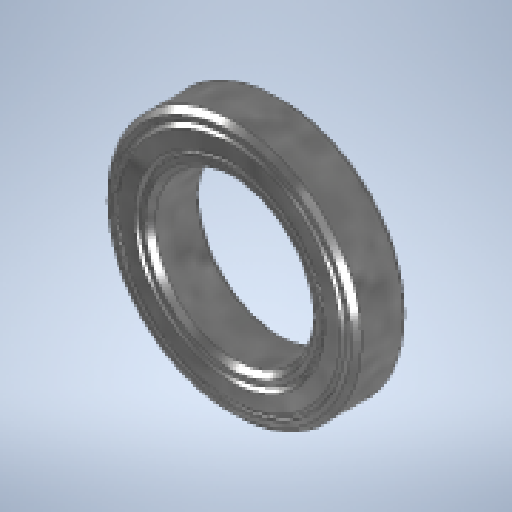
# Autodesk Inventor part: 6203베어링
Saved by Autodesk Inventor 2023 (Build 270158000, 158)
## iProperties
Created: 2022-06-08
Part Number: 6203베어링
Material: 일반
Document SubType Name: Modeling
Designer: fly01
Density: 1 g/cm^3
Appearance: 기본값
Author: fly01
Autodesk Inventor part; units mm, degrees
ref_plane "YZ Plane" through (0, 0, 0) normal (1, 0, 0) x (0, 1, 0)
ref_plane "XZ Plane" through (0, 0, 0) normal (0, 1, 0) x (-1, 0, 0)
ref_plane "XY Plane" through (0, 0, 0) normal (0, 0, 1) x (1, 0, 0)
sketch "스케치1" plane through (0, 0, 0) normal (0, 0, 1) x (1, 0, 0)
  circle A0 centre (0, 0) radius 7.5
  circle A1 centre (0, 0) radius 12
  dimension "d0" = 15
  dimension "d1" = 24
  constraints: 2 centre point, 2 coincident
  measures "d0" diameter of A0
  measures "d1" diameter of A1
extrude "돌출1" add sketch "스케치1" along normal mid plane 5
chamfer "모따기1" distance 0.5 angle 45 4 edges at (-12, 0, 2.5) (-12, 0, -2.5) (-7.5, 0, 2.5) (-7.5, 0, -2.5)
sketch "스케치2" plane through (0, 0, 0) normal (0, 1, 0) x (-1, 0, 0)
  line L0 (-11.5, 2.5) -> (11.5, 2.5) projected
  line L1 (11, 2.5) -> (11, 2.2414)
  line L2 (10.8293, 2.1707) -> (10.5, 2.5)
  line L3 (12, 0) -> (7.5, 0)
  line L4 (7.5, 2) -> (7.5, -2) projected
  arc A0 (10.8293, 2.1707) -> (11, 2.2414) centre (10.9, 2.2414) ccw
  line L5 (9.75, 0) -> (9.75, 1.7292)
  line L6 (8.5, 2.5) -> (8.5, 2.2414)
  line L7 (8.6707, 2.1707) -> (9, 2.5)
  arc A1 (8.5, 2.2414) -> (8.6707, 2.1707) centre (8.6, 2.2414) ccw
  line L8 (11, -2.5) -> (11, -2.2414)
  line L9 (10.8293, -2.1707) -> (10.5, -2.5)
  arc A2 (11, -2.2414) -> (10.8293, -2.1707) centre (10.9, -2.2414) ccw
  line L10 (8.5, -2.5) -> (8.5, -2.2414)
  line L11 (8.6707, -2.1707) -> (9, -2.5)
  arc A3 (8.6707, -2.1707) -> (8.5, -2.2414) centre (8.6, -2.2414) ccw
  line L12 (0, 0) -> (0, -13.1586)
  line L13 (11.5, -2.5) -> (-11.5, -2.5) projected
  line L14 (12, -2) -> (12, 2) projected
  point P0 (11, 2)
  point P1 (8, 2.5)
  point P2 (8.5, 2)
  point P3 (11, -2)
  point P4 (8, -2.5)
  point P5 (8.5, -2)
  dimension "d7" = 0.5
  dimension "d8" = 0.5
  dimension "d9" = 0.5
  dimension "d10" = 0.1
  constraints: 22 end point, 21 symmetric about line, 10 point on line, 8 point on circle, 4 centre point, 3 midpoint, 3 vertical, 2 tangent, 3 other
  measures "d7" distance of L0.end L1.start
  measures "d8" distance of L1.start point (11, 2)
  measures "d9" distance of L1.start L2.end
  measures "d10" radius of A0
revolve "회전1" cut sketch "스케치2" angle 360 about axis through (0, 0, 0) along (0, 0, -1)
